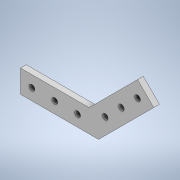
# Autodesk Inventor part: 1x3 V plate
Saved by Autodesk Inventor 2020 (Build 240168000, 168)
## iProperties
Created: 2020-01-28
Part Number: 1x3 V plate
Material: Generic
Document SubType Name: Modeling
Designer: 339294
Density: 1 g/cm^3
Appearance: Default
Author: 339294
Autodesk Inventor part; units mm, degrees
ref_plane "YZ Plane" through (0, 0, 0) normal (1, 0, 0) x (0, 1, 0)
ref_plane "XZ Plane" through (0, 0, 0) normal (0, 1, 0) x (-1, 0, 0)
ref_plane "XY Plane" through (0, 0, 0) normal (0, 0, 1) x (1, 0, 0)
sketch "Sketch1" plane through (0, 0, 0) normal (0, 0, 1) x (1, 0, 0)
  line L0 (0, 0) -> (0, 25.4)
  line L1 (0, 25.4) -> (76.2, 25.4)
  line L2 (76.2, 25.4) -> (130.0815, 79.2815)
  line L3 (130.0815, 79.2815) -> (148.042, 61.321)
  line L4 (148.042, 61.321) -> (86.721, 0)
  line L5 (86.721, 0) -> (0, 0)
  circle A0 centre (12.7, 12.7) radius 3.2512
  circle A1 centre (38.1, 12.7) radius 3.2512
  circle A2 centre (63.5, 12.7) radius 3.2512
  circle A3 centre (130.0815, 61.321) radius 3.2512
  circle A4 centre (112.121, 43.3605) radius 3.2512
  circle A5 centre (94.1605, 25.4) radius 3.2512
  dimension "d0" = 25.4
  dimension "d1" = 76.2
  dimension "d2" = 76.2
  dimension "d3" = 135
  dimension "d4" = 25.4
  dimension "d5" = 6.5024
  dimension "d6" = 12.7
  dimension "d9" = 25.4
  dimension "d14" = 12.7
  dimension "d15" = 6.5024
  dimension "d16" = 12.7
  dimension "d17" = 12.7
  dimension "d23" = 25.4
  constraints: 12 end point, 6 centre point, 3 perpendicular, 1 horizontal, 1 parallel, 1 vertical, 9 other
  measures "d0" distance of L0.start L0.end
  measures "d1" distance of L0.end L1.end
  measures "d2" distance of L1.end L2.end
  measures "d3" angle of L2 L1
  measures "d4" distance of L2.end L3.end
  measures "d5" diameter of A0
  measures "d6" distance from line of L0 A0.centre
  measures "d9" distance of A0.centre A1.centre
  measures "d14" distance from line of L1 A0.centre
  measures "d15" diameter of A3
  measures "d16" distance from line of L3 A3.centre
  measures "d17" distance from line of L2 A3.centre
  measures "d23" distance of A3.centre A4.centre
extrude "Extrusion1" add sketch "Sketch1" along normal blind 6.35
body "Solid1"
